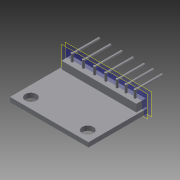
# Autodesk Inventor part: accelerometer
Saved by Autodesk Inventor 2016 (Build 200138000, 138)
## iProperties
Created: 2015-11-17
Part Number: accelerometer
Material: Generic
Document SubType Name: Modeling
Designer: Jufo
Density: 1 g/cm^3
Appearance: Default
Author: Jufo
Autodesk Inventor part; units mm, degrees
ref_plane "YZ Plane" through (0, 0, 0) normal (1, 0, 0) x (0, 1, 0)
ref_plane "XZ Plane" through (0, 0, 0) normal (0, 1, 0) x (-1, 0, 0)
ref_plane "XY Plane" through (0, 0, 0) normal (0, 0, 1) x (1, 0, 0)
sketch "Sketch1" plane through (0, 0, 0) normal (0, 1, 0) x (-1, 0, 0)
  line L0 (25.8895, 13.6798) -> (4.8895, 13.6798)
  line L1 (4.8895, 13.6798) -> (4.8895, -2.1202)
  line L2 (4.8895, -2.1202) -> (25.8895, -2.1202)
  line L3 (25.8895, -2.1202) -> (25.8895, 13.6798)
  circle A0 centre (22.9895, 10.9798) radius 1.5
  circle A1 centre (7.7895, 10.9798) radius 1.5
  point P0 (0, 0)
  dimension "d0" = 21
  dimension "d1" = 15.8
  dimension "d2" = 3
  dimension "d3" = 3
  dimension "d4" = 2.9
  dimension "d5" = 2.9
  dimension "d6" = 2.7
  dimension "d7" = 2.7
  constraints: 8 end point, 2 centre point, 2 parallel, 1 horizontal, 1 perpendicular
  measures "d0" distance of L2.end L1.end
  measures "d1" distance of L1.end L0.end
  measures "d2" diameter of A0
  measures "d3" diameter of A1
  measures "d4" distance from line of L1 A1.centre
  measures "d5" distance from line of L3 A0.centre
  measures "d6" distance from line of L0 A0.centre
  measures "d7" distance from line of L0 A1.centre
extrude "Extrusion1" add sketch "Sketch1" along normal blind 1.2
sketch "Sketch2" plane through (0, 1.2, 0) normal (0, 1, 0) x (1, 0, 0)
  line L0 (-5.3895, 2.1202) -> (-25.3895, 2.1202)
  line L1 (-25.3895, 2.1202) -> (-25.3895, -0.3798)
  line L2 (-25.3895, -0.3798) -> (-5.3895, -0.3798)
  line L3 (-5.3895, -0.3798) -> (-5.3895, 2.1202)
  line L4 (-4.8895, 2.1202) -> (-25.8895, 2.1202) projected
  line L5 (-4.8895, -13.6798) -> (-4.8895, 2.1202) projected
  point P0 (0, 0)
  dimension "d10" = 20
  dimension "d11" = 2.5
  dimension "d12" = 0
  dimension "d13" = 0.5
  constraints: 8 end point, 2 parallel, 1 horizontal, 1 perpendicular
  measures "d10" distance of L2.end L1.end
  measures "d11" distance of L0.end L1.end
  measures "d12" distance between parallel lines of L4 L0
  measures "d13" distance between parallel lines of L5 L3
extrude "Extrusion2" add sketch "Sketch2" along normal blind 2
sketch "Sketch3" plane through (0, 3.2, 0) normal (0, 1, 0) x (1, 0, 0)
  circle A0 centre (-6.9895, 0.8702) radius 0.3
  circle A1 centre (-9.3895, 0.8702) radius 0.3
  circle A2 centre (-11.7895, 0.8702) radius 0.3
  circle A3 centre (-14.7895, 0.8702) radius 0.3
  circle A4 centre (-17.7895, 0.8702) radius 0.3
  circle A5 centre (-20.7895, 0.8702) radius 0.3
  circle A6 centre (-23.7895, 0.8702) radius 0.3
  line L0 (-5.3895, -0.3798) -> (-5.3895, 2.1202) projected
  point P0 (0, 0)
  dimension "d16" = 0.6
  dimension "d17" = 0.6
  dimension "d18" = 0.6
  dimension "d19" = 0.6
  dimension "d20" = 0.6
  dimension "d21" = 0.6
  dimension "d22" = 0.6
  dimension "d24" = 1.6
  dimension "d25" = 3
  dimension "d26" = 3
  dimension "d27" = 3
  dimension "d28" = 3
  dimension "d29" = 3
  dimension "d30" = 3
  constraints: 7 centre point
  measures "d16" diameter of A0
  measures "d17" diameter of A1
  measures "d18" diameter of A2
  measures "d19" diameter of A3
  measures "d20" diameter of A4
  measures "d21" diameter of A5
  measures "d22" diameter of A6
  measures "d24" distance from line of A0.centre L0
  measures "d27" distance between centres of A3 A2
  measures "d28" distance between centres of A4 A3
  measures "d29" distance between centres of A5 A4
  measures "d30" distance between centres of A6 A5
extrude "Extrusion3" add sketch "Sketch3" along normal blind 2
ref_plane "Work Plane2" through (-5.3895, 3.2, -0.6202) normal (0, 0, -1) x (-1, 0, 0)
ref_plane "Work Plane1" through (-5.3895, 3.2, -2.1202) normal (0, 0, -1) x (-1, 0, 0)
sketch "Sketch4" plane through (-5.3895, 3.2, -0.6202) normal (0, 0, -1) x (-1, 0, 0)
  line L0 (1.9, 2) -> (1.3, 2) projected
  circle A0 centre (4, 1.7) radius 0.3
  circle A1 centre (6.4, 1.7) radius 0.3
  circle A2 centre (9.4, 1.7) radius 0.3
  circle A3 centre (1.6, 1.7) radius 0.3
  circle A4 centre (12.4, 1.7) radius 0.3
  circle A5 centre (15.4, 1.7) radius 0.3
  circle A6 centre (18.4, 1.7) radius 0.3
  point P0 (-5.3895, -3.2)
  dimension "d37" = 0.6
  dimension "d38" = 0.6
  dimension "d39" = 0.6
  dimension "d40" = 0.6
  dimension "d41" = 0.6
  dimension "d42" = 0.6
  dimension "d43" = 0.6
  constraints: 7 centre point
  measures "d37" diameter of A0
  measures "d38" diameter of A1
  measures "d39" diameter of A2
  measures "d40" diameter of A3
  measures "d41" diameter of A4
  measures "d42" diameter of A5
  measures "d43" diameter of A6
extrude "Extrusion4" add sketch "Sketch4" along normal blind 7.5
equation "\"d7\" = d6"
body "Solid1"
